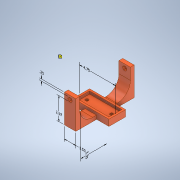
# Autodesk Inventor part: connectorToTubeBrackeCradleTmp
Saved by Autodesk Inventor 2022 (Build 260153070, 153G)
## iProperties
Created: 2020-07-23
Part Number: connectorToTubeBrackeCradleTmp
Material: PBT Plastic
Document SubType Name: Modeling
Designer: robst
Density: 1.31 g/cm^3
Appearance: Smooth - Light Orange
Mass: 391.418 g
Surface Area: 592.905 cm^2
Volume: 298.793 cm^3
Author: robst
Autodesk Inventor part; units mm, degrees
(part 1 of 3)
ref_plane "YZ Plane" through (0, 0, 0) normal (1, 0, 0) x (0, 1, 0)
ref_plane "XZ Plane" through (0, 0, 0) normal (0, 1, 0) x (-1, 0, 0)
ref_plane "XY Plane" through (0, 0, 0) normal (0, 0, 1) x (1, 0, 0)
sketch "Sketch1" plane through (0, 0, 0) normal (0, 1, 0) x (-1, 0, 0)
  line L0 (53.975, 21.59) -> (-53.975, 21.59)
  line L1 (-53.975, 21.59) -> (-53.975, -21.59)
  line L2 (-53.975, -21.59) -> (53.975, -21.59)
  line L3 (53.975, -21.59) -> (53.975, 21.59)
  line L4 (53.975, 21.59) -> (-53.975, -21.59) construction
  line L5 (-53.975, 21.59) -> (53.975, -21.59) construction
  line L6 (60.325, 27.94) -> (-60.325, 27.94)
  line L7 (-60.325, 27.94) -> (-60.325, -27.94)
  line L8 (-60.325, -27.94) -> (60.325, -27.94)
  line L9 (60.325, -27.94) -> (60.325, 27.94)
  line L10 (60.325, 27.94) -> (-60.325, -27.94) construction
  line L11 (-60.325, 27.94) -> (60.325, -27.94) construction
  point P0 (0, 0)
  dimension "d0" = 43.18
  dimension "d1" = 107.95
  dimension "d2" = 6.35
  dimension "d3" = 6.35
  constraints: 24 end point, 4 midpoint, 4 parallel, 2 horizontal, 2 perpendicular
  measures "d0" distance of L0.end L1.end
  measures "d1" distance between parallel lines of L1 L3
  measures "d2" distance between parallel lines of L8 L2
  measures "d3" distance between parallel lines of L9 L3
extrude "Extrusion1" add sketch "Sketch1" against normal blind 12.065 contours L3 L2 L1 L0 | L9 L8 L7 L6
extrude "Extrusion2" add sketch "Sketch1" along normal blind 8.89
sketch "Sketch2" plane through (0, 0, 0) normal (0, 1, 0) x (1, 0, 0)
  line L0 (-53.975, 21.59) -> (-53.975, -21.59) construction
  line L1 (-53.975, 0) -> (53.975, 0) construction
  line L2 (53.975, -21.59) -> (53.975, 21.59) construction
  point P0 (0, 0)
  point P1 (-41.275, 0)
  point P2 (41.275, 0)
  dimension "d8" = 12.7
  dimension "d9" = 12.7
  constraints: 2 end point, 2 midpoint, 2 point on line
  measures "d8" distance from line of point (-41.275, 0) L0
  measures "d9" distance from line of point (41.275, 0) L2
hole "Hole1" at (-41.275, 0, 0) at (41.275, 0, 0) direction (0, -1, 0) diameter 5.1054 end through all counterbore diameter 10.16 counterbore depth 2.54 clearance for "Hex Machine Screw" size "#10" standard "Ansi Unified Screw Threads"
sketch "Sketch15" plane through (-60.325, -12.065, 27.94) normal (0, 0, 1) x (1, 0, 0)
  line L0 (0, 20.955) -> (120.65, 20.955) projected
  line L1 (120.65, 20.955) -> (120.65, 0) projected
  line L2 (120.65, 0) -> (0, 0) projected
  line L3 (0, 0) -> (0, 20.955) projected
  line L4 (0, 20.955) -> (120.65, 0) construction
  line L5 (0, 0) -> (120.65, 20.955) construction
  line L6 (41.275, 0) -> (79.375, 0)
  line L7 (79.375, 0) -> (79.375, 20.955)
  line L8 (79.375, 20.955) -> (41.275, 20.955)
  line L9 (41.275, 20.955) -> (41.275, 0)
  line L10 (41.275, 0) -> (79.375, 20.955) construction
  line L11 (79.375, 0) -> (41.275, 20.955) construction
  line L12 (114.3, 12.065) -> (6.35, 12.065) projected
  point P0 (60.325, 12.065)
  point P1 (60.325, 10.4775)
  point P2 (79.375, 12.065)
  point P3 (41.275, 12.065)
  point P4 (41.275, 0)
  point P5 (79.375, 0)
  dimension "d109" = 38.1
  constraints: 16 end point, 3 midpoint, 3 parallel, 1 collinear, 1 perpendicular
  measures "d109" distance between parallel lines of L7 L9
extrude "Extrusion10" add sketch "Sketch15" along normal blind 69.85 contours L12 L7 L2 L9
sketch "Sketch16" plane through (-19.05, 0, 27.94) normal (0, 1, 0) x (1, 0, 0)
  line L0 (0, -69.85) -> (38.1, -69.85) projected
  line L1 (38.1, 0) -> (38.1, -69.85) projected
  line L2 (0, -69.85) -> (38.1, -69.85)
  line L3 (38.1, -69.85) -> (38.1, -57.15)
  line L4 (38.1, -57.15) -> (0, -57.15)
  line L5 (0, -57.15) -> (0, -69.85)
  point P0 (19.05, 27.94)
  dimension "d103" = 12.7
  constraints: 8 end point, 2 parallel, 1 horizontal, 1 perpendicular, 1 point on line
  measures "d103" distance between parallel lines of L4 L0
extrude "Extrusion11" add sketch "Sketch16" along normal blind 82.55
sketch "Sketch17" plane through (-60.325, -12.065, 97.79) normal (0, 0, 1) x (1, 0, 0)
  line L0 (41.275, 94.615) -> (79.375, 94.615) construction
  line L1 (41.275, 0) -> (79.375, 0) construction
  line L2 (79.375, 94.615) -> (41.275, 94.615) construction
  line L3 (60.325, 94.615) -> (60.325, 0) construction
  line L4 (67.804, 81.915) -> (64.0645, 75.438)
  line L5 (64.0645, 75.438) -> (56.5855, 75.438)
  line L6 (56.5855, 75.438) -> (52.846, 81.915)
  line L7 (52.846, 81.915) -> (56.5855, 88.392)
  line L8 (56.5855, 88.392) -> (64.0645, 88.392)
  line L9 (64.0645, 88.392) -> (67.804, 81.915)
  point P0 (60.325, 12.065)
  point P1 (60.325, 81.915)
  dimension "d119" = 12.7
  dimension "d120" = 12.954
  constraints: 14 end point, 2 midpoint, 1 horizontal, 1 point on line, 13 other
  measures "d119" distance from line of point (60.325, 81.915) L0
  measures "d120" distance between parallel lines of L5 L8
extrude "Extrusion12" cut sketch "Sketch17" against normal through all
mirror "Mirror8" about plane through (0, 0, 0) normal (0, 0, 1) of "Extrusion11", "Extrusion12", "Extrusion10"
fillet "Fillet1" radius 44.45 2 edges at (0, 0, -85.09) (0, 0, 85.09)
sketch "Sketch18" plane through (0, -12.065, 0) normal (0, -1, 0) x (1, 0, 0)
  line L0 (-19.05, 97.79) -> (19.05, 97.79) construction
  line L1 (0, 97.79) -> (0, -97.79) construction
  line L2 (-19.05, -97.79) -> (19.05, -97.79) construction
  line L3 (-6.35, -88.0484) -> (-6.35, -88.8511)
  line L4 (-6.35, -88.8511) -> (-6.8337, -88.8511)
  spline S0 degree 2 poles (-6.8337, -88.8511) (-6.6793, -89.0364) (-6.4735, -89.3091) (-6.386, -89.4943) knots 0 0 0 1 2 2 2
  spline S1 degree 2 poles (-6.386, -89.4943) (-6.3037, -89.6642) (-6.2162, -90.0295) (-6.2162, -90.2714) knots 0 0 0 1 2 2 2
  spline S2 degree 2 poles (-6.2162, -90.2714) (-6.2162, -90.6625) (-6.5404, -91.3211) (-6.8543, -91.5527) knots 0 0 0 1 2 2 2
  spline S3 degree 2 poles (-6.8543, -91.5527) (-7.1682, -91.7843) (-8.0944, -92.0415) (-8.6965, -92.0415) knots 0 0 0 1 2 2 2
  spline S4 degree 2 poles (-8.6965, -92.0415) (-9.3243, -92.0415) (-10.2403, -91.7174) (-10.585, -91.4343) knots 0 0 0 1 2 2 2
  spline S5 degree 2 poles (-10.585, -91.4343) (-10.8938, -91.1719) (-11.2489, -90.436) (-11.2489, -90.0295) knots 0 0 0 1 2 2 2
  spline S6 degree 2 poles (-11.2489, -90.0295) (-11.2489, -89.6744) (-11.0893, -89.1444) (-10.9247, -88.8511) knots 0 0 0 1 2 2 2
  line L5 (-10.9247, -88.8511) -> (-12.983, -88.8511)
  line L6 (-12.983, -88.8511) -> (-12.983, -88.0484)
  line L7 (-12.983, -88.0484) -> (-6.35, -88.0484)
  line L8 (-7.5078, -88.8511) -> (-10.2609, -88.8511)
  spline S7 degree 2 poles (-10.2609, -88.8511) (-10.4049, -89.1496) (-10.513, -89.623) (-10.513, -89.8957) knots 0 0 0 1 2 2 2
  spline S8 degree 2 poles (-10.513, -89.8957) (-10.513, -90.5132) (-9.5868, -91.2131) (-8.712, -91.2131) knots 0 0 0 1 2 2 2
  spline S9 degree 2 poles (-8.712, -91.2131) (-7.868, -91.2131) (-6.9778, -90.6779) (-6.9778, -90.0861) knots 0 0 0 1 2 2 2
  spline S10 degree 2 poles (-6.9778, -90.0861) (-6.9778, -89.7722) (-7.266, -89.1341) (-7.5078, -88.8511) knots 0 0 0 1 2 2 2
  line L9 (-6.35, -86.0672) -> (-6.35, -86.8699)
  line L10 (-6.35, -86.8699) -> (-11.1151, -86.8699)
  line L11 (-11.1151, -86.8699) -> (-11.1151, -86.0672)
  line L12 (-11.1151, -86.0672) -> (-6.35, -86.0672)
  line L13 (-11.9075, -86.0106) -> (-11.9075, -86.9214)
  line L14 (-11.9075, -86.9214) -> (-12.7412, -86.9214)
  line L15 (-12.7412, -86.9214) -> (-12.7412, -86.0106)
  line L16 (-12.7412, -86.0106) -> (-11.9075, -86.0106)
  line L17 (-10.2557, -82.3622) -> (-10.2557, -82.4033)
  spline S11 degree 2 poles (-10.2557, -82.4033) (-10.2814, -82.496) (-10.2917, -82.6966) (-10.2917, -82.8356) knots 0 0 0 1 2 2 2
  spline S12 degree 2 poles (-10.2917, -82.8356) (-10.2917, -83.1598) (-10.0087, -83.7979) (-9.7308, -84.086) knots 0 0 0 1 2 2 2
  line L18 (-9.7308, -84.086) -> (-6.35, -84.086)
  line L19 (-6.35, -84.086) -> (-6.35, -84.8888)
  line L20 (-6.35, -84.8888) -> (-11.1151, -84.8888)
  line L21 (-11.1151, -84.8888) -> (-11.1151, -84.086)
  line L22 (-11.1151, -84.086) -> (-10.4049, -84.086)
  spline S13 degree 2 poles (-10.4049, -84.086) (-10.796, -83.6486) (-11.1151, -82.9951) (-11.1151, -82.6864) knots 0 0 0 1 2 2 2
  spline S14 degree 2 poles (-11.1151, -82.6864) (-11.1151, -82.5629) (-11.1048, -82.4394) (-11.0893, -82.3622) knots 0 0 0 1 2 2 2
  line L23 (-11.0893, -82.3622) -> (-10.2557, -82.3622)
  line L24 (-6.35, -80.2678) -> (-6.35, -81.2867)
  line L25 (-6.35, -81.2867) -> (-7.5644, -81.2867)
  line L26 (-7.5644, -81.2867) -> (-7.5644, -80.2678)
  line L27 (-7.5644, -80.2678) -> (-6.35, -80.2678)
  line L28 (-9.9006, -80.2678) -> (-9.9006, -81.2867)
  line L29 (-9.9006, -81.2867) -> (-11.1151, -81.2867)
  line L30 (-11.1151, -81.2867) -> (-11.1151, -80.2678)
  line L31 (-11.1151, -80.2678) -> (-9.9006, -80.2678)
  line L32 (-6.35, -74.3809) -> (-11.9487, -74.3809)
  line L33 (-11.9487, -74.3809) -> (-11.9487, -76.5113)
  line L34 (-11.9487, -76.5113) -> (-12.7, -76.5113)
  line L35 (-12.7, -76.5113) -> (-12.7, -71.4066)
  line L36 (-12.7, -71.4066) -> (-11.9487, -71.4066)
  line L37 (-11.9487, -71.4066) -> (-11.9487, -73.537)
  line L38 (-11.9487, -73.537) -> (-6.35, -73.537)
  line L39 (-6.35, -73.537) -> (-6.35, -74.3809)
  spline S15 degree 2 poles (-6.2419, -68.7514) (-6.2419, -69.8937) (-7.5233, -71.1493) (-8.7068, -71.1493) knots 0 0 0 1 2 2 2
  spline S16 degree 2 poles (-8.7068, -71.1493) (-9.8698, -71.1493) (-11.2489, -69.9298) (-11.2489, -68.9469) knots 0 0 0 1 2 2 2
  spline S17 degree 2 poles (-11.2489, -68.9469) (-11.2489, -68.5043) (-10.9916, -67.8199) (-10.7188, -67.5678) knots 0 0 0 1 2 2 2
  spline S18 degree 2 poles (-10.7188, -67.5678) (-10.4461, -67.3105) (-9.6588, -67.0378) (-9.0876, -67.0378) knots 0 0 0 1 2 2 2
  line L40 (-9.0876, -67.0378) -> (-8.6502, -67.0378)
  line L41 (-8.6502, -67.0378) -> (-8.6502, -70.3363)
  spline S19 degree 2 poles (-8.6502, -70.3363) (-7.8217, -70.3363) (-6.9418, -69.5026) (-6.9418, -68.7616) knots 0 0 0 1 2 2 2
  spline S20 degree 2 poles (-6.9418, -68.7616) (-6.9418, -68.4992) (-7.0601, -67.9898) (-7.1528, -67.7839) knots 0 0 0 1 2 2 2
  spline S21 degree 2 poles (-7.1528, -67.7839) (-7.2557, -67.5678) (-7.4358, -67.2693) (-7.5181, -67.1716) knots 0 0 0 1 2 2 2
  line L42 (-7.5181, -67.1716) -> (-7.5181, -67.1253)
  line L43 (-7.5181, -67.1253) -> (-6.6433, -67.1253)
  spline S22 degree 2 poles (-6.6433, -67.1253) (-6.5867, -67.2642) (-6.422, -67.6862) (-6.3757, -67.8508) knots 0 0 0 1 2 2 2
  spline S23 degree 2 poles (-6.3757, -67.8508) (-6.3088, -68.0824) (-6.2419, -68.4632) (-6.2419, -68.7514) knots 0 0 0 1 2 2 2
  spline S24 degree 2 poles (-9.2626, -67.8199) (-9.5868, -67.8302) (-10.0602, -67.964) (-10.2197, -68.0927) knots 0 0 0 1 2 2 2
  spline S25 degree 2 poles (-10.2197, -68.0927) (-10.3998, -68.2316) (-10.5902, -68.669) (-10.5902, -68.9932) knots 0 0 0 1 2 2 2
  spline S26 degree 2 poles (-10.5902, -68.9932) (-10.5902, -69.3123) (-10.3998, -69.7599) (-10.2145, -69.9452) knots 0 0 0 1 2 2 2
  spline S27 degree 2 poles (-10.2145, -69.9452) (-10.0241, -70.1253) (-9.5662, -70.3105) (-9.2626, -70.3363) knots 0 0 0 1 2 2 2
  line L44 (-9.2626, -70.3363) -> (-9.2626, -67.8199)
  line L45 (-6.35, -65.4065) -> (-6.35, -66.2093)
  line L46 (-6.35, -66.2093) -> (-12.983, -66.2093)
  line L47 (-12.983, -66.2093) -> (-12.983, -65.4065)
  line L48 (-12.983, -65.4065) -> (-6.35, -65.4065)
  spline S28 degree 2 poles (-6.2419, -62.1595) (-6.2419, -63.3019) (-7.5233, -64.5575) (-8.7068, -64.5575) knots 0 0 0 1 2 2 2
  spline S29 degree 2 poles (-8.7068, -64.5575) (-9.8698, -64.5575) (-11.2489, -63.3379) (-11.2489, -62.355) knots 0 0 0 1 2 2 2
  spline S30 degree 2 poles (-11.2489, -62.355) (-11.2489, -61.9125) (-10.9916, -61.2281) (-10.7188, -60.9759) knots 0 0 0 1 2 2 2
  spline S31 degree 2 poles (-10.7188, -60.9759) (-10.4461, -60.7187) (-9.6588, -60.4459) (-9.0876, -60.4459) knots 0 0 0 1 2 2 2
  line L49 (-9.0876, -60.4459) -> (-8.6502, -60.4459)
  line L50 (-8.6502, -60.4459) -> (-8.6502, -63.7444)
  spline S32 degree 2 poles (-8.6502, -63.7444) (-7.8217, -63.7444) (-6.9418, -62.9108) (-6.9418, -62.1698) knots 0 0 0 1 2 2 2
  spline S33 degree 2 poles (-6.9418, -62.1698) (-6.9418, -61.9073) (-7.0601, -61.3979) (-7.1528, -61.1921) knots 0 0 0 1 2 2 2
  spline S34 degree 2 poles (-7.1528, -61.1921) (-7.2557, -60.9759) (-7.4358, -60.6775) (-7.5181, -60.5797) knots 0 0 0 1 2 2 2
  line L51 (-7.5181, -60.5797) -> (-7.5181, -60.5334)
  line L52 (-7.5181, -60.5334) -> (-6.6433, -60.5334)
  spline S35 degree 2 poles (-6.6433, -60.5334) (-6.5867, -60.6723) (-6.422, -61.0943) (-6.3757, -61.259) knots 0 0 0 1 2 2 2
  spline S36 degree 2 poles (-6.3757, -61.259) (-6.3088, -61.4905) (-6.2419, -61.8713) (-6.2419, -62.1595) knots 0 0 0 1 2 2 2
  spline S37 degree 2 poles (-9.2626, -61.2281) (-9.5868, -61.2384) (-10.0602, -61.3722) (-10.2197, -61.5008) knots 0 0 0 1 2 2 2
  spline S38 degree 2 poles (-10.2197, -61.5008) (-10.3998, -61.6398) (-10.5902, -62.0772) (-10.5902, -62.4014) knots 0 0 0 1 2 2 2
  spline S39 degree 2 poles (-10.5902, -62.4014) (-10.5902, -62.7204) (-10.3998, -63.1681) (-10.2145, -63.3533) knots 0 0 0 1 2 2 2
  spline S40 degree 2 poles (-10.2145, -63.3533) (-10.0241, -63.5334) (-9.5662, -63.7187) (-9.2626, -63.7444) knots 0 0 0 1 2 2 2
  line L53 (-9.2626, -63.7444) -> (-9.2626, -61.2281)
  spline S41 degree 2 poles (-6.2368, -58.3464) (-6.2368, -58.825) (-6.4941, -59.6535) (-6.6382, -59.9262) knots 0 0 0 1 2 2 2
  line L54 (-6.6382, -59.9262) -> (-7.5387, -59.9262)
  line L55 (-7.5387, -59.9262) -> (-7.5387, -59.885)
  spline S42 degree 2 poles (-7.5387, -59.885) (-7.4564, -59.7821) (-7.2608, -59.5042) (-7.1528, -59.2727) knots 0 0 0 1 2 2 2
  spline S43 degree 2 poles (-7.1528, -59.2727) (-7.055, -59.072) (-6.9109, -58.578) (-6.9109, -58.3155) knots 0 0 0 1 2 2 2
  spline S44 degree 2 poles (-6.9109, -58.3155) (-6.9109, -58.1251) (-6.9984, -57.6877) (-7.0704, -57.5848) knots 0 0 0 1 2 2 2
  spline S45 degree 2 poles (-7.0704, -57.5848) (-7.1682, -57.4356) (-7.3895, -57.3018) (-7.6159, -57.3018) knots 0 0 0 1 2 2 2
  spline S46 degree 2 poles (-7.6159, -57.3018) (-7.8989, -57.3018) (-8.1922, -57.6105) (-8.29, -58.0068) knots 0 0 0 1 2 2 2
  spline S47 degree 2 poles (-8.29, -58.0068) (-8.326, -58.1612) (-8.4289, -58.6552) (-8.4855, -58.8661) knots 0 0 0 1 2 2 2
  spline S48 degree 2 poles (-8.4855, -58.8661) (-8.6451, -59.4116) (-9.3037, -59.9056) (-9.772, -59.9056) knots 0 0 0 1 2 2 2
  spline S49 degree 2 poles (-9.772, -59.9056) (-10.4204, -59.9056) (-11.2283, -58.933) (-11.2283, -58.1303) knots 0 0 0 1 2 2 2
  spline S50 degree 2 poles (-11.2283, -58.1303) (-11.2283, -57.7341) (-11.0327, -56.9313) (-10.8835, -56.6586) knots 0 0 0 1 2 2 2
  line L56 (-10.8835, -56.6586) -> (-10.0241, -56.6586)
  line L57 (-10.0241, -56.6586) -> (-10.0241, -56.6997)
  spline S51 degree 2 poles (-10.0241, -56.6997) (-10.2712, -57.0085) (-10.5542, -57.7598) (-10.5542, -58.1457) knots 0 0 0 1 2 2 2
  spline S52 degree 2 poles (-10.5542, -58.1457) (-10.5542, -58.542) (-10.2197, -59.0874) (-9.8852, -59.0874) knots 0 0 0 1 2 2 2
  spline S53 degree 2 poles (-9.8852, -59.0874) (-9.5816, -59.0874) (-9.2883, -58.7632) (-9.1957, -58.403) knots 0 0 0 1 2 2 2
  spline S54 degree 2 poles (-9.1957, -58.403) (-9.1494, -58.2281) (-9.0567, -57.7855) (-9.0001, -57.5437) knots 0 0 0 1 2 2 2
  spline S55 degree 2 poles (-9.0001, -57.5437) (-8.8663, -57.0188) (-8.254, -56.4836) (-7.7239, -56.4836) knots 0 0 0 1 2 2 2
  spline S56 degree 2 poles (-7.7239, -56.4836) (-7.4152, -56.4836) (-6.8697, -56.7255) (-6.669, -56.9622) knots 0 0 0 1 2 2 2
  spline S57 degree 2 poles (-6.669, -56.9622) (-6.4581, -57.2143) (-6.2368, -57.8576) (-6.2368, -58.3464) knots 0 0 0 1 2 2 2
  spline S58 degree 2 poles (-6.2419, -53.8438) (-6.2419, -54.3378) (-6.5455, -55.156) (-6.8543, -55.4493) knots 0 0 0 1 2 2 2
  spline S59 degree 2 poles (-6.8543, -55.4493) (-7.1579, -55.7426) (-8.0944, -56.0668) (-8.7222, -56.0668) knots 0 0 0 1 2 2 2
  spline S60 degree 2 poles (-8.7222, -56.0668) (-9.35, -56.0668) (-10.266, -55.7323) (-10.5748, -55.4493) knots 0 0 0 1 2 2 2
  spline S61 degree 2 poles (-10.5748, -55.4493) (-10.8887, -55.1663) (-11.2231, -54.3275) (-11.2231, -53.8438) knots 0 0 0 1 2 2 2
  spline S62 degree 2 poles (-11.2231, -53.8438) (-11.2231, -53.4527) (-11.0019, -52.722) (-10.8578, -52.439) knots 0 0 0 1 2 2 2
  line L58 (-10.8578, -52.439) -> (-9.9573, -52.439)
  line L59 (-9.9573, -52.439) -> (-9.9573, -52.4853)
  spline S63 degree 2 poles (-9.9573, -52.4853) (-10.0293, -52.5727) (-10.2145, -52.8403) (-10.3123, -53.0307) knots 0 0 0 1 2 2 2
  spline S64 degree 2 poles (-10.3123, -53.0307) (-10.3947, -53.2005) (-10.5233, -53.6534) (-10.5233, -53.8592) knots 0 0 0 1 2 2 2
  spline S65 degree 2 poles (-10.5233, -53.8592) (-10.5233, -54.4819) (-9.5816, -55.2383) (-8.7222, -55.2383) knots 0 0 0 1 2 2 2
  spline S66 degree 2 poles (-8.7222, -55.2383) (-7.8835, -55.2383) (-6.9418, -54.5076) (-6.9418, -53.8592) knots 0 0 0 1 2 2 2
  spline S67 degree 2 poles (-6.9418, -53.8592) (-6.9418, -53.4681) (-7.266, -52.758) (-7.5181, -52.4853) knots 0 0 0 1 2 2 2
  line L60 (-7.5181, -52.4853) -> (-7.5181, -52.439)
  line L61 (-7.5181, -52.439) -> (-6.6176, -52.439)
  spline S68 degree 2 poles (-6.6176, -52.439) (-6.561, -52.5573) (-6.4015, -52.9175) (-6.3654, -53.0616) knots 0 0 0 1 2 2 2
  spline S69 degree 2 poles (-6.3654, -53.0616) (-6.3037, -53.2674) (-6.2419, -53.5916) (-6.2419, -53.8438) knots 0 0 0 1 2 2 2
  spline S70 degree 2 poles (-8.7325, -47.7922) (-7.5284, -47.7922) (-6.2162, -48.9501) (-6.2162, -49.9175) knots 0 0 0 1 2 2 2
  spline S71 degree 2 poles (-6.2162, -49.9175) (-6.2162, -50.9106) (-7.5696, -52.0479) (-8.7325, -52.0479) knots 0 0 0 1 2 2 2
  spline S72 degree 2 poles (-8.7325, -52.0479) (-9.9264, -52.0479) (-11.2489, -50.8746) (-11.2489, -49.9175) knots 0 0 0 1 2 2 2
  spline S73 degree 2 poles (-11.2489, -49.9175) (-11.2489, -48.9501) (-9.9315, -47.7922) (-8.7325, -47.7922) knots 0 0 0 1 2 2 2
  spline S74 degree 2 poles (-8.7325, -48.6207) (-9.6588, -48.6207) (-10.5593, -49.2948) (-10.5593, -49.9175) knots 0 0 0 1 2 2 2
  spline S75 degree 2 poles (-10.5593, -49.9175) (-10.5593, -50.5401) (-9.6588, -51.2194) (-8.7325, -51.2194) knots 0 0 0 1 2 2 2
  spline S76 degree 2 poles (-8.7325, -51.2194) (-7.832, -51.2194) (-6.9058, -50.5401) (-6.9058, -49.9175) knots 0 0 0 1 2 2 2
  spline S77 degree 2 poles (-6.9058, -49.9175) (-6.9058, -49.3) (-7.8166, -48.6207) (-8.7325, -48.6207) knots 0 0 0 1 2 2 2
  spline S78 degree 2 poles (-8.8612, -42.9757) (-7.6673, -42.9757) (-6.2574, -44.1129) (-6.2574, -44.9826) knots 0 0 0 1 2 2 2
  spline S79 degree 2 poles (-6.2574, -44.9826) (-6.2574, -45.3377) (-6.422, -45.8831) (-6.5919, -46.1661) knots 0 0 0 1 2 2 2
  line L62 (-6.5919, -46.1661) -> (-4.5953, -46.1661)
  line L63 (-4.5953, -46.1661) -> (-4.5953, -46.9689)
  line L64 (-4.5953, -46.9689) -> (-11.1151, -46.9689)
  line L65 (-11.1151, -46.9689) -> (-11.1151, -46.1661)
  line L66 (-11.1151, -46.1661) -> (-10.6159, -46.1661)
  spline S80 degree 2 poles (-10.6159, -46.1661) (-10.8887, -45.8677) (-11.2489, -45.137) (-11.2489, -44.7099) knots 0 0 0 1 2 2 2
  spline S81 degree 2 poles (-11.2489, -44.7099) (-11.2489, -43.8917) (-9.9521, -42.9757) (-8.8612, -42.9757) knots 0 0 0 1 2 2 2
  spline S82 degree 2 poles (-8.7686, -43.8042) (-9.5868, -43.8042) (-10.4873, -44.3239) (-10.4873, -44.9054) knots 0 0 0 1 2 2 2
  spline S83 degree 2 poles (-10.4873, -44.9054) (-10.4873, -45.245) (-10.1837, -45.8831) (-9.947, -46.1661) knots 0 0 0 1 2 2 2
  line L67 (-9.947, -46.1661) -> (-7.2402, -46.1661)
  spline S84 degree 2 poles (-7.2402, -46.1661) (-7.091, -45.8522) (-6.9778, -45.4046) (-6.9778, -45.1164) knots 0 0 0 1 2 2 2
  spline S85 degree 2 poles (-6.9778, -45.1164) (-6.9778, -44.4937) (-7.8938, -43.8042) (-8.7686, -43.8042) knots 0 0 0 1 2 2 2
  spline S86 degree 2 poles (-6.2419, -40.0734) (-6.2419, -41.2158) (-7.5233, -42.4714) (-8.7068, -42.4714) knots 0 0 0 1 2 2 2
  spline S87 degree 2 poles (-8.7068, -42.4714) (-9.8698, -42.4714) (-11.2489, -41.2518) (-11.2489, -40.269) knots 0 0 0 1 2 2 2
  spline S88 degree 2 poles (-11.2489, -40.269) (-11.2489, -39.8264) (-10.9916, -39.142) (-10.7188, -38.8899) knots 0 0 0 1 2 2 2
  spline S89 degree 2 poles (-10.7188, -38.8899) (-10.4461, -38.6326) (-9.6588, -38.3599) (-9.0876, -38.3599) knots 0 0 0 1 2 2 2
  line L68 (-9.0876, -38.3599) -> (-8.6502, -38.3599)
  line L69 (-8.6502, -38.3599) -> (-8.6502, -41.6584)
  spline S90 degree 2 poles (-8.6502, -41.6584) (-7.8217, -41.6584) (-6.9418, -40.8247) (-6.9418, -40.0837) knots 0 0 0 1 2 2 2
  spline S91 degree 2 poles (-6.9418, -40.0837) (-6.9418, -39.8213) (-7.0601, -39.3118) (-7.1528, -39.106) knots 0 0 0 1 2 2 2
  spline S92 degree 2 poles (-7.1528, -39.106) (-7.2557, -38.8899) (-7.4358, -38.5914) (-7.5181, -38.4937) knots 0 0 0 1 2 2 2
  line L70 (-7.5181, -38.4937) -> (-7.5181, -38.4473)
  line L71 (-7.5181, -38.4473) -> (-6.6433, -38.4473)
  spline S93 degree 2 poles (-6.6433, -38.4473) (-6.5867, -38.5863) (-6.422, -39.0082) (-6.3757, -39.1729) knots 0 0 0 1 2 2 2
  spline S94 degree 2 poles (-6.3757, -39.1729) (-6.3088, -39.4045) (-6.2419, -39.7853) (-6.2419, -40.0734) knots 0 0 0 1 2 2 2
  spline S95 degree 2 poles (-9.2626, -39.142) (-9.5868, -39.1523) (-10.0602, -39.2861) (-10.2197, -39.4148) knots 0 0 0 1 2 2 2
  spline S96 degree 2 poles (-10.2197, -39.4148) (-10.3998, -39.5537) (-10.5902, -39.9911) (-10.5902, -40.3153) knots 0 0 0 1 2 2 2
  spline S97 degree 2 poles (-10.5902, -40.3153) (-10.5902, -40.6343) (-10.3998, -41.082) (-10.2145, -41.2673) knots 0 0 0 1 2 2 2
  spline S98 degree 2 poles (-10.2145, -41.2673) (-10.0241, -41.4474) (-9.5662, -41.6326) (-9.2626, -41.6584) knots 0 0 0 1 2 2 2
  line L72 (-9.2626, -41.6584) -> (-9.2626, -39.142)
  spline S99 degree 2 poles (-10.7857, -33.4713) (-10.3741, -33.4713) (-9.6331, -33.7646) (-9.3758, -34.027) knots 0 0 0 1 2 2 2
  spline S100 degree 2 poles (-9.3758, -34.027) (-9.0516, -34.3564) (-8.7171, -35.2466) (-8.7171, -35.9259) knots 0 0 0 1 2 2 2
  line L73 (-8.7171, -35.9259) -> (-8.7171, -36.6411)
  line L74 (-8.7171, -36.6411) -> (-6.35, -36.6411)
  line L75 (-6.35, -36.6411) -> (-6.35, -37.4851)
  line L76 (-6.35, -37.4851) -> (-12.7, -37.4851)
  line L77 (-12.7, -37.4851) -> (-12.7, -35.8898)
  spline S101 degree 2 poles (-12.7, -35.8898) (-12.7, -35.3238) (-12.5147, -34.5313) (-12.3038, -34.2277) knots 0 0 0 1 2 2 2
  spline S102 degree 2 poles (-12.3038, -34.2277) (-12.0619, -33.8727) (-11.3158, -33.4713) (-10.7857, -33.4713) knots 0 0 0 1 2 2 2
  spline S103 degree 2 poles (-10.76, -34.3512) (-11.0893, -34.3512) (-11.5731, -34.5776) (-11.7274, -34.8092) knots 0 0 0 1 2 2 2
  spline S104 degree 2 poles (-11.7274, -34.8092) (-11.8612, -35.0099) (-11.9693, -35.5451) (-11.9693, -35.9413) knots 0 0 0 1 2 2 2
  line L78 (-11.9693, -35.9413) -> (-11.9693, -36.6411)
  line L79 (-11.9693, -36.6411) -> (-9.4375, -36.6411)
  line L80 (-9.4375, -36.6411) -> (-9.4375, -36.0648)
  spline S105 degree 2 poles (-9.4375, -36.0648) (-9.4375, -35.5502) (-9.6022, -34.9173) (-9.8183, -34.7114) knots 0 0 0 1 2 2 2
  spline S106 degree 2 poles (-9.8183, -34.7114) (-10.0087, -34.521) (-10.4564, -34.3512) (-10.76, -34.3512) knots 0 0 0 1 2 2 2
  line L81 (-10.2557, -30.2037) -> (-10.2557, -30.2448)
  spline S107 degree 2 poles (-10.2557, -30.2448) (-10.2814, -30.3375) (-10.2917, -30.5381) (-10.2917, -30.6771) knots 0 0 0 1 2 2 2
  spline S108 degree 2 poles (-10.2917, -30.6771) (-10.2917, -31.0013) (-10.0087, -31.6394) (-9.7308, -31.9275) knots 0 0 0 1 2 2 2
  line L82 (-9.7308, -31.9275) -> (-6.35, -31.9275)
  line L83 (-6.35, -31.9275) -> (-6.35, -32.7303)
  line L84 (-6.35, -32.7303) -> (-11.1151, -32.7303)
  line L85 (-11.1151, -32.7303) -> (-11.1151, -31.9275)
  line L86 (-11.1151, -31.9275) -> (-10.4049, -31.9275)
  spline S109 degree 2 poles (-10.4049, -31.9275) (-10.796, -31.4901) (-11.1151, -30.8366) (-11.1151, -30.5279) knots 0 0 0 1 2 2 2
  spline S110 degree 2 poles (-11.1151, -30.5279) (-11.1151, -30.4044) (-11.1048, -30.2808) (-11.0893, -30.2037) knots 0 0 0 1 2 2 2
  line L87 (-11.0893, -30.2037) -> (-10.2557, -30.2037)
  spline S111 degree 2 poles (-8.7325, -25.665) (-7.5284, -25.665) (-6.2162, -26.8228) (-6.2162, -27.7903) knots 0 0 0 1 2 2 2
  spline S112 degree 2 poles (-6.2162, -27.7903) (-6.2162, -28.7834) (-7.5696, -29.9206) (-8.7325, -29.9206) knots 0 0 0 1 2 2 2
  spline S113 degree 2 poles (-8.7325, -29.9206) (-9.9264, -29.9206) (-11.2489, -28.7474) (-11.2489, -27.7903) knots 0 0 0 1 2 2 2
  spline S114 degree 2 poles (-11.2489, -27.7903) (-11.2489, -26.8228) (-9.9315, -25.665) (-8.7325, -25.665) knots 0 0 0 1 2 2 2
  spline S115 degree 2 poles (-8.7325, -26.4935) (-9.6588, -26.4935) (-10.5593, -27.1676) (-10.5593, -27.7903) knots 0 0 0 1 2 2 2
  spline S116 degree 2 poles (-10.5593, -27.7903) (-10.5593, -28.4129) (-9.6588, -29.0922) (-8.7325, -29.0922) knots 0 0 0 1 2 2 2
  spline S117 degree 2 poles (-8.7325, -29.0922) (-7.832, -29.0922) (-6.9058, -28.4129) (-6.9058, -27.7903) knots 0 0 0 1 2 2 2
  spline S118 degree 2 poles (-6.9058, -27.7903) (-6.9058, -27.1727) (-7.8166, -26.4935) (-8.7325, -26.4935) knots 0 0 0 1 2 2 2
  spline S119 degree 2 poles (-6.2162, -23.5449) (-5.4032, -23.5449) (-4.5489, -24.4197) (-4.5489, -25.1864) knots 0 0 0 1 2 2 2
  spline S120 degree 2 poles (-4.5489, -25.1864) (-4.5489, -25.3202) (-4.5747, -25.6496) (-4.6004, -25.8091) knots 0 0 0 1 2 2 2
  line L88 (-4.6004, -25.8091) -> (-5.3208, -25.8091)
  line L89 (-5.3208, -25.8091) -> (-5.3208, -25.7628)
  spline S121 degree 2 poles (-5.3208, -25.7628) (-5.3002, -25.6702) (-5.2591, -25.4437) (-5.2591, -25.3408) knots 0 0 0 1 2 2 2
  spline S122 degree 2 poles (-5.2591, -25.3408) (-5.2591, -25.0218) (-5.4186, -24.605) (-5.5884, -24.5072) knots 0 0 0 1 2 2 2
  spline S123 degree 2 poles (-5.5884, -24.5072) (-5.7428, -24.4094) (-6.2111, -24.3477) (-6.5455, -24.3477) knots 0 0 0 1 2 2 2
  line L90 (-6.5455, -24.3477) -> (-10.4513, -24.3477)
  line L91 (-10.4513, -24.3477) -> (-10.4513, -25.207)
  line L92 (-10.4513, -25.207) -> (-11.1151, -25.207)
  line L93 (-11.1151, -25.207) -> (-11.1151, -23.5449)
  line L94 (-11.1151, -23.5449) -> (-6.2162, -23.5449)
  line L95 (-11.9075, -23.5398) -> (-11.9075, -24.4506)
  line L96 (-11.9075, -24.4506) -> (-12.7412, -24.4506)
  line L97 (-12.7412, -24.4506) -> (-12.7412, -23.5398)
  line L98 (-12.7412, -23.5398) -> (-11.9075, -23.5398)
  spline S124 degree 2 poles (-6.2419, -20.3133) (-6.2419, -21.4557) (-7.5233, -22.7113) (-8.7068, -22.7113) knots 0 0 0 1 2 2 2
  spline S125 degree 2 poles (-8.7068, -22.7113) (-9.8698, -22.7113) (-11.2489, -21.4917) (-11.2489, -20.5088) knots 0 0 0 1 2 2 2
  spline S126 degree 2 poles (-11.2489, -20.5088) (-11.2489, -20.0663) (-10.9916, -19.3819) (-10.7188, -19.1298) knots 0 0 0 1 2 2 2
  spline S127 degree 2 poles (-10.7188, -19.1298) (-10.4461, -18.8725) (-9.6588, -18.5997) (-9.0876, -18.5997) knots 0 0 0 1 2 2 2
  line L99 (-9.0876, -18.5997) -> (-8.6502, -18.5997)
  line L100 (-8.6502, -18.5997) -> (-8.6502, -21.8982)
  spline S128 degree 2 poles (-8.6502, -21.8982) (-7.8217, -21.8982) (-6.9418, -21.0646) (-6.9418, -20.3236) knots 0 0 0 1 2 2 2
  spline S129 degree 2 poles (-6.9418, -20.3236) (-6.9418, -20.0612) (-7.0601, -19.5517) (-7.1528, -19.3459) knots 0 0 0 1 2 2 2
  spline S130 degree 2 poles (-7.1528, -19.3459) (-7.2557, -19.1298) (-7.4358, -18.8313) (-7.5181, -18.7335) knots 0 0 0 1 2 2 2
  line L101 (-7.5181, -18.7335) -> (-7.5181, -18.6872)
  line L102 (-7.5181, -18.6872) -> (-6.6433, -18.6872)
  spline S131 degree 2 poles (-6.6433, -18.6872) (-6.5867, -18.8262) (-6.422, -19.2481) (-6.3757, -19.4128) knots 0 0 0 1 2 2 2
  spline S132 degree 2 poles (-6.3757, -19.4128) (-6.3088, -19.6443) (-6.2419, -20.0251) (-6.2419, -20.3133) knots 0 0 0 1 2 2 2
  spline S133 degree 2 poles (-9.2626, -19.3819) (-9.5868, -19.3922) (-10.0602, -19.526) (-10.2197, -19.6546) knots 0 0 0 1 2 2 2
  spline S134 degree 2 poles (-10.2197, -19.6546) (-10.3998, -19.7936) (-10.5902, -20.231) (-10.5902, -20.5552) knots 0 0 0 1 2 2 2
  spline S135 degree 2 poles (-10.5902, -20.5552) (-10.5902, -20.8742) (-10.3998, -21.3219) (-10.2145, -21.5071) knots 0 0 0 1 2 2 2
  spline S136 degree 2 poles (-10.2145, -21.5071) (-10.0241, -21.6873) (-9.5662, -21.8725) (-9.2626, -21.8982) knots 0 0 0 1 2 2 2
  line L103 (-9.2626, -21.8982) -> (-9.2626, -19.3819)
  spline S137 degree 2 poles (-6.2419, -15.893) (-6.2419, -16.387) (-6.5455, -17.2052) (-6.8543, -17.4985) knots 0 0 0 1 2 2 2
  spline S138 degree 2 poles (-6.8543, -17.4985) (-7.1579, -17.7918) (-8.0944, -18.116) (-8.7222, -18.116) knots 0 0 0 1 2 2 2
  spline S139 degree 2 poles (-8.7222, -18.116) (-9.35, -18.116) (-10.266, -17.7815) (-10.5748, -17.4985) knots 0 0 0 1 2 2 2
  spline S140 degree 2 poles (-10.5748, -17.4985) (-10.8887, -17.2155) (-11.2231, -16.3767) (-11.2231, -15.893) knots 0 0 0 1 2 2 2
  spline S141 degree 2 poles (-11.2231, -15.893) (-11.2231, -15.5019) (-11.0019, -14.7712) (-10.8578, -14.4882) knots 0 0 0 1 2 2 2
  line L104 (-10.8578, -14.4882) -> (-9.9573, -14.4882)
  line L105 (-9.9573, -14.4882) -> (-9.9573, -14.5345)
  spline S142 degree 2 poles (-9.9573, -14.5345) (-10.0293, -14.622) (-10.2145, -14.8896) (-10.3123, -15.08) knots 0 0 0 1 2 2 2
  spline S143 degree 2 poles (-10.3123, -15.08) (-10.3947, -15.2498) (-10.5233, -15.7026) (-10.5233, -15.9084) knots 0 0 0 1 2 2 2
  spline S144 degree 2 poles (-10.5233, -15.9084) (-10.5233, -16.5311) (-9.5816, -17.2875) (-8.7222, -17.2875) knots 0 0 0 1 2 2 2
  spline S145 degree 2 poles (-8.7222, -17.2875) (-7.8835, -17.2875) (-6.9418, -16.5568) (-6.9418, -15.9084) knots 0 0 0 1 2 2 2
  spline S146 degree 2 poles (-6.9418, -15.9084) (-6.9418, -15.5174) (-7.266, -14.8072) (-7.5181, -14.5345) knots 0 0 0 1 2 2 2
  line L106 (-7.5181, -14.5345) -> (-7.5181, -14.4882)
  line L107 (-7.5181, -14.4882) -> (-6.6176, -14.4882)
  spline S147 degree 2 poles (-6.6176, -14.4882) (-6.561, -14.6065) (-6.4015, -14.9667) (-6.3654, -15.1108) knots 0 0 0 1 2 2 2
  spline S148 degree 2 poles (-6.3654, -15.1108) (-6.3037, -15.3167) (-6.2419, -15.6409) (-6.2419, -15.893) knots 0 0 0 1 2 2 2
  spline S149 degree 2 poles (-6.2574, -12.3166) (-6.2574, -12.9702) (-7.0035, -13.706) (-7.8114, -13.706) knots 0 0 0 1 2 2 2
  line L108 (-7.8114, -13.706) -> (-10.4513, -13.706)
  line L109 (-10.4513, -13.706) -> (-10.4513, -14.2463)
  line L110 (-10.4513, -14.2463) -> (-11.1151, -14.2463)
  line L111 (-11.1151, -14.2463) -> (-11.1151, -13.706)
  line L112 (-11.1151, -13.706) -> (-12.4839, -13.706)
  line L113 (-12.4839, -13.706) -> (-12.4839, -12.9033)
  line L114 (-12.4839, -12.9033) -> (-11.1151, -12.9033)
  line L115 (-11.1151, -12.9033) -> (-11.1151, -11.4264)
  line L116 (-11.1151, -11.4264) -> (-10.4513, -11.4264)
  line L117 (-10.4513, -11.4264) -> (-10.4513, -12.9033)
  line L118 (-10.4513, -12.9033) -> (-8.1819, -12.9033)
  spline S150 degree 2 poles (-8.1819, -12.9033) (-7.8217, -12.9033) (-7.4255, -12.8775) (-7.2557, -12.79) knots 0 0 0 1 2 2 2
  spline S151 degree 2 poles (-7.2557, -12.79) (-7.1064, -12.718) (-6.9572, -12.3938) (-6.9572, -12.1159) knots 0 0 0 1 2 2 2
  spline S152 degree 2 poles (-6.9572, -12.1159) (-6.9572, -11.9204) (-7.0756, -11.555) (-7.1116, -11.4727) knots 0 0 0 1 2 2 2
  line L119 (-7.1116, -11.4727) -> (-7.1116, -11.4264)
  line L120 (-7.1116, -11.4264) -> (-6.3912, -11.4264)
  spline S153 degree 2 poles (-6.3912, -11.4264) (-6.3294, -11.6528) (-6.2574, -12.1159) (-6.2574, -12.3166) knots 0 0 0 1 2 2 2
  spline S154 degree 2 poles (-6.2368, -9.5482) (-6.2368, -10.0267) (-6.4941, -10.8552) (-6.6382, -11.1279) knots 0 0 0 1 2 2 2
  line L121 (-6.6382, -11.1279) -> (-7.5387, -11.1279)
  line L122 (-7.5387, -11.1279) -> (-7.5387, -11.0868)
  spline S155 degree 2 poles (-7.5387, -11.0868) (-7.4564, -10.9838) (-7.2608, -10.706) (-7.1528, -10.4744) knots 0 0 0 1 2 2 2
  spline S156 degree 2 poles (-7.1528, -10.4744) (-7.055, -10.2737) (-6.9109, -9.7797) (-6.9109, -9.5173) knots 0 0 0 1 2 2 2
  spline S157 degree 2 poles (-6.9109, -9.5173) (-6.9109, -9.3269) (-6.9984, -8.8895) (-7.0704, -8.7866) knots 0 0 0 1 2 2 2
  spline S158 degree 2 poles (-7.0704, -8.7866) (-7.1682, -8.6373) (-7.3895, -8.5035) (-7.6159, -8.5035) knots 0 0 0 1 2 2 2
  spline S159 degree 2 poles (-7.6159, -8.5035) (-7.8989, -8.5035) (-8.1922, -8.8123) (-8.29, -9.2085) knots 0 0 0 1 2 2 2
  spline S160 degree 2 poles (-8.29, -9.2085) (-8.326, -9.3629) (-8.4289, -9.8569) (-8.4855, -10.0679) knots 0 0 0 1 2 2 2
  spline S161 degree 2 poles (-8.4855, -10.0679) (-8.6451, -10.6133) (-9.3037, -11.1073) (-9.772, -11.1073) knots 0 0 0 1 2 2 2
  spline S162 degree 2 poles (-9.772, -11.1073) (-10.4204, -11.1073) (-11.2283, -10.1348) (-11.2283, -9.332) knots 0 0 0 1 2 2 2
  spline S163 degree 2 poles (-11.2283, -9.332) (-11.2283, -8.9358) (-11.0327, -8.133) (-10.8835, -7.8603) knots 0 0 0 1 2 2 2
  line L123 (-10.8835, -7.8603) -> (-10.0241, -7.8603)
  line L124 (-10.0241, -7.8603) -> (-10.0241, -7.9015)
  spline S164 degree 2 poles (-10.0241, -7.9015) (-10.2712, -8.2102) (-10.5542, -8.9615) (-10.5542, -9.3475) knots 0 0 0 1 2 2 2
  spline S165 degree 2 poles (-10.5542, -9.3475) (-10.5542, -9.7437) (-10.2197, -10.2892) (-9.8852, -10.2892) knots 0 0 0 1 2 2 2
  spline S166 degree 2 poles (-9.8852, -10.2892) (-9.5816, -10.2892) (-9.2883, -9.965) (-9.1957, -9.6048) knots 0 0 0 1 2 2 2
  spline S167 degree 2 poles (-9.1957, -9.6048) (-9.1494, -9.4298) (-9.0567, -8.9873) (-9.0001, -8.7454) knots 0 0 0 1 2 2 2
  spline S168 degree 2 poles (-9.0001, -8.7454) (-8.8663, -8.2205) (-8.254, -7.6853) (-7.7239, -7.6853) knots 0 0 0 1 2 2 2
  spline S169 degree 2 poles (-7.7239, -7.6853) (-7.4152, -7.6853) (-6.8697, -7.9272) (-6.669, -8.1639) knots 0 0 0 1 2 2 2
  spline S170 degree 2 poles (-6.669, -8.1639) (-6.4581, -8.4161) (-6.2368, -9.0593) (-6.2368, -9.5482) knots 0 0 0 1 2 2 2
  line L125 (-4.9709, -4.0935) -> (-4.9709, -4.814)
  line L126 (-4.9709, -4.814) -> (-12.983, -7.2994)
  line L127 (-12.983, -7.2994) -> (-12.983, -6.5687)
  line L128 (-12.983, -6.5687) -> (-4.9709, -4.0935)
  line L129 (-6.35, -2.0558) -> (-11.9487, -2.0558)
  line L130 (-11.9487, -2.0558) -> (-11.9487, -4.1862)
  line L131 (-11.9487, -4.1862) -> (-12.7, -4.1862)
  line L132 (-12.7, -4.1862) -> (-12.7, 0.9185)
  line L133 (-12.7, 0.9185) -> (-11.9487, 0.9185)
  line L134 (-11.9487, 0.9185) -> (-11.9487, -1.2118)
  line L135 (-11.9487, -1.2118) -> (-6.35, -1.2118)
  line L136 (-6.35, -1.2118) -> (-6.35, -2.0558)
  spline S171 degree 2 poles (-6.2419, 3.5738) (-6.2419, 2.4314) (-7.5233, 1.1758) (-8.7068, 1.1758) knots 0 0 0 1 2 2 2
  spline S172 degree 2 poles (-8.7068, 1.1758) (-9.8698, 1.1758) (-11.2489, 2.3954) (-11.2489, 3.3783) knots 0 0 0 1 2 2 2
  spline S173 degree 2 poles (-11.2489, 3.3783) (-11.2489, 3.8208) (-10.9916, 4.5052) (-10.7188, 4.7574) knots 0 0 0 1 2 2 2
  spline S174 degree 2 poles (-10.7188, 4.7574) (-10.4461, 5.0147) (-9.6588, 5.2874) (-9.0876, 5.2874) knots 0 0 0 1 2 2 2
  line L137 (-9.0876, 5.2874) -> (-8.6502, 5.2874)
  line L138 (-8.6502, 5.2874) -> (-8.6502, 1.9889)
  spline S175 degree 2 poles (-8.6502, 1.9889) (-7.8217, 1.9889) (-6.9418, 2.8225) (-6.9418, 3.5635) knots 0 0 0 1 2 2 2
  spline S176 degree 2 poles (-6.9418, 3.5635) (-6.9418, 3.826) (-7.0601, 4.3354) (-7.1528, 4.5412) knots 0 0 0 1 2 2 2
  spline S177 degree 2 poles (-7.1528, 4.5412) (-7.2557, 4.7574) (-7.4358, 5.0558) (-7.5181, 5.1536) knots 0 0 0 1 2 2 2
  line L139 (-7.5181, 5.1536) -> (-7.5181, 5.1999)
  line L140 (-7.5181, 5.1999) -> (-6.6433, 5.1999)
  spline S178 degree 2 poles (-6.6433, 5.1999) (-6.5867, 5.061) (-6.422, 4.639) (-6.3757, 4.4743) knots 0 0 0 1 2 2 2
  spline S179 degree 2 poles (-6.3757, 4.4743) (-6.3088, 4.2428) (-6.2419, 3.862) (-6.2419, 3.5738) knots 0 0 0 1 2 2 2
  spline S180 degree 2 poles (-9.2626, 4.5052) (-9.5868, 4.4949) (-10.0602, 4.3611) (-10.2197, 4.2325) knots 0 0 0 1 2 2 2
  spline S181 degree 2 poles (-10.2197, 4.2325) (-10.3998, 4.0935) (-10.5902, 3.6561) (-10.5902, 3.332) knots 0 0 0 1 2 2 2
  spline S182 degree 2 poles (-10.5902, 3.332) (-10.5902, 3.0129) (-10.3998, 2.5652) (-10.2145, 2.38) knots 0 0 0 1 2 2 2
  spline S183 degree 2 poles (-10.2145, 2.38) (-10.0241, 2.1999) (-9.5662, 2.0146) (-9.2626, 1.9889) knots 0 0 0 1 2 2 2
  line L141 (-9.2626, 1.9889) -> (-9.2626, 4.5052)
  line L142 (-6.35, 6.9186) -> (-6.35, 6.1159)
  line L143 (-6.35, 6.1159) -> (-12.983, 6.1159)
  line L144 (-12.983, 6.1159) -> (-12.983, 6.9186)
  line L145 (-12.983, 6.9186) -> (-6.35, 6.9186)
  spline S184 degree 2 poles (-6.2419, 10.1657) (-6.2419, 9.0233) (-7.5233, 7.7677) (-8.7068, 7.7677) knots 0 0 0 1 2 2 2
  spline S185 degree 2 poles (-8.7068, 7.7677) (-9.8698, 7.7677) (-11.2489, 8.9873) (-11.2489, 9.9701) knots 0 0 0 1 2 2 2
  spline S186 degree 2 poles (-11.2489, 9.9701) (-11.2489, 10.4127) (-10.9916, 11.0971) (-10.7188, 11.3492) knots 0 0 0 1 2 2 2
  spline S187 degree 2 poles (-10.7188, 11.3492) (-10.4461, 11.6065) (-9.6588, 11.8792) (-9.0876, 11.8792) knots 0 0 0 1 2 2 2
  line L146 (-9.0876, 11.8792) -> (-8.6502, 11.8792)
  line L147 (-8.6502, 11.8792) -> (-8.6502, 8.5807)
  spline S188 degree 2 poles (-8.6502, 8.5807) (-7.8217, 8.5807) (-6.9418, 9.4144) (-6.9418, 10.1554) knots 0 0 0 1 2 2 2
  spline S189 degree 2 poles (-6.9418, 10.1554) (-6.9418, 10.4178) (-7.0601, 10.9273) (-7.1528, 11.1331) knots 0 0 0 1 2 2 2
  spline S190 degree 2 poles (-7.1528, 11.1331) (-7.2557, 11.3492) (-7.4358, 11.6477) (-7.5181, 11.7454) knots 0 0 0 1 2 2 2
  line L148 (-7.5181, 11.7454) -> (-7.5181, 11.7918)
  line L149 (-7.5181, 11.7918) -> (-6.6433, 11.7918)
  spline S191 degree 2 poles (-6.6433, 11.7918) (-6.5867, 11.6528) (-6.422, 11.2309) (-6.3757, 11.0662) knots 0 0 0 1 2 2 2
  spline S192 degree 2 poles (-6.3757, 11.0662) (-6.3088, 10.8346) (-6.2419, 10.4538) (-6.2419, 10.1657) knots 0 0 0 1 2 2 2
  spline S193 degree 2 poles (-9.2626, 11.0971) (-9.5868, 11.0868) (-10.0602, 10.953) (-10.2197, 10.8243) knots 0 0 0 1 2 2 2
  spline S194 degree 2 poles (-10.2197, 10.8243) (-10.3998, 10.6854) (-10.5902, 10.248) (-10.5902, 9.9238) knots 0 0 0 1 2 2 2
  spline S195 degree 2 poles (-10.5902, 9.9238) (-10.5902, 9.6048) (-10.3998, 9.1571) (-10.2145, 8.9718) knots 0 0 0 1 2 2 2
  spline S196 degree 2 poles (-10.2145, 8.9718) (-10.0241, 8.7917) (-9.5662, 8.6065) (-9.2626, 8.5807) knots 0 0 0 1 2 2 2
  line L150 (-9.2626, 8.5807) -> (-9.2626, 11.0971)
  spline S197 degree 2 poles (-6.2368, 13.9788) (-6.2368, 13.5002) (-6.4941, 12.6717) (-6.6382, 12.399) knots 0 0 0 1 2 2 2
  line L151 (-6.6382, 12.399) -> (-7.5387, 12.399)
  line L152 (-7.5387, 12.399) -> (-7.5387, 12.4401)
  spline S198 degree 2 poles (-7.5387, 12.4401) (-7.4564, 12.5431) (-7.2608, 12.8209) (-7.1528, 13.0525) knots 0 0 0 1 2 2 2
  spline S199 degree 2 poles (-7.1528, 13.0525) (-7.055, 13.2532) (-6.9109, 13.7472) (-6.9109, 14.0096) knots 0 0 0 1 2 2 2
  spline S200 degree 2 poles (-6.9109, 14.0096) (-6.9109, 14.2) (-6.9984, 14.6374) (-7.0704, 14.7403) knots 0 0 0 1 2 2 2
  spline S201 degree 2 poles (-7.0704, 14.7403) (-7.1682, 14.8896) (-7.3895, 15.0234) (-7.6159, 15.0234) knots 0 0 0 1 2 2 2
  spline S202 degree 2 poles (-7.6159, 15.0234) (-7.8989, 15.0234) (-8.1922, 14.7146) (-8.29, 14.3184) knots 0 0 0 1 2 2 2
  spline S203 degree 2 poles (-8.29, 14.3184) (-8.326, 14.164) (-8.4289, 13.67) (-8.4855, 13.459) knots 0 0 0 1 2 2 2
  spline S204 degree 2 poles (-8.4855, 13.459) (-8.6451, 12.9136) (-9.3037, 12.4196) (-9.772, 12.4196) knots 0 0 0 1 2 2 2
  spline S205 degree 2 poles (-9.772, 12.4196) (-10.4204, 12.4196) (-11.2283, 13.3921) (-11.2283, 14.1949) knots 0 0 0 1 2 2 2
  spline S206 degree 2 poles (-11.2283, 14.1949) (-11.2283, 14.5911) (-11.0327, 15.3939) (-10.8835, 15.6666) knots 0 0 0 1 2 2 2
  line L153 (-10.8835, 15.6666) -> (-10.0241, 15.6666)
  line L154 (-10.0241, 15.6666) -> (-10.0241, 15.6254)
  spline S207 degree 2 poles (-10.0241, 15.6254) (-10.2712, 15.3167) (-10.5542, 14.5654) (-10.5542, 14.1794) knots 0 0 0 1 2 2 2
  spline S208 degree 2 poles (-10.5542, 14.1794) (-10.5542, 13.7832) (-10.2197, 13.2377) (-9.8852, 13.2377) knots 0 0 0 1 2 2 2
  spline S209 degree 2 poles (-9.8852, 13.2377) (-9.5816, 13.2377) (-9.2883, 13.5619) (-9.1957, 13.9221) knots 0 0 0 1 2 2 2
  spline S210 degree 2 poles (-9.1957, 13.9221) (-9.1494, 14.0971) (-9.0567, 14.5397) (-9.0001, 14.7815) knots 0 0 0 1 2 2 2
  spline S211 degree 2 poles (-9.0001, 14.7815) (-8.8663, 15.3064) (-8.254, 15.8416) (-7.7239, 15.8416) knots 0 0 0 1 2 2 2
  spline S212 degree 2 poles (-7.7239, 15.8416) (-7.4152, 15.8416) (-6.8697, 15.5997) (-6.669, 15.363) knots 0 0 0 1 2 2 2
  spline S213 degree 2 poles (-6.669, 15.363) (-6.4581, 15.1108) (-6.2368, 14.4676) (-6.2368, 13.9788) knots 0 0 0 1 2 2 2
  spline S214 degree 2 poles (-6.2419, 18.4814) (-6.2419, 17.9874) (-6.5455, 17.1692) (-6.8543, 16.8759) knots 0 0 0 1 2 2 2
  spline S215 degree 2 poles (-6.8543, 16.8759) (-7.1579, 16.5826) (-8.0944, 16.2584) (-8.7222, 16.2584) knots 0 0 0 1 2 2 2
  spline S216 degree 2 poles (-8.7222, 16.2584) (-9.35, 16.2584) (-10.266, 16.5929) (-10.5748, 16.8759) knots 0 0 0 1 2 2 2
  spline S217 degree 2 poles (-10.5748, 16.8759) (-10.8887, 17.1589) (-11.2231, 17.9977) (-11.2231, 18.4814) knots 0 0 0 1 2 2 2
  spline S218 degree 2 poles (-11.2231, 18.4814) (-11.2231, 18.8725) (-11.0019, 19.6032) (-10.8578, 19.8862) knots 0 0 0 1 2 2 2
  line L155 (-10.8578, 19.8862) -> (-9.9573, 19.8862)
  line L156 (-9.9573, 19.8862) -> (-9.9573, 19.8399)
  spline S219 degree 2 poles (-9.9573, 19.8399) (-10.0293, 19.7524) (-10.2145, 19.4848) (-10.3123, 19.2944) knots 0 0 0 1 2 2 2
  spline S220 degree 2 poles (-10.3123, 19.2944) (-10.3947, 19.1246) (-10.5233, 18.6718) (-10.5233, 18.4659) knots 0 0 0 1 2 2 2
  spline S221 degree 2 poles (-10.5233, 18.4659) (-10.5233, 17.8433) (-9.5816, 17.0869) (-8.7222, 17.0869) knots 0 0 0 1 2 2 2
  spline S222 degree 2 poles (-8.7222, 17.0869) (-7.8835, 17.0869) (-6.9418, 17.8176) (-6.9418, 18.4659) knots 0 0 0 1 2 2 2
  spline S223 degree 2 poles (-6.9418, 18.4659) (-6.9418, 18.857) (-7.266, 19.5672) (-7.5181, 19.8399) knots 0 0 0 1 2 2 2
  line L157 (-7.5181, 19.8399) -> (-7.5181, 19.8862)
  line L158 (-7.5181, 19.8862) -> (-6.6176, 19.8862)
  spline S224 degree 2 poles (-6.6176, 19.8862) (-6.561, 19.7679) (-6.4015, 19.4076) (-6.3654, 19.2636) knots 0 0 0 1 2 2 2
  spline S225 degree 2 poles (-6.3654, 19.2636) (-6.3037, 19.0577) (-6.2419, 18.7335) (-6.2419, 18.4814) knots 0 0 0 1 2 2 2
  spline S226 degree 2 poles (-8.7325, 24.5329) (-7.5284, 24.5329) (-6.2162, 23.3751) (-6.2162, 22.4077) knots 0 0 0 1 2 2 2
  spline S227 degree 2 poles (-6.2162, 22.4077) (-6.2162, 21.4145) (-7.5696, 20.2773) (-8.7325, 20.2773) knots 0 0 0 1 2 2 2
  spline S228 degree 2 poles (-8.7325, 20.2773) (-9.9264, 20.2773) (-11.2489, 21.4505) (-11.2489, 22.4077) knots 0 0 0 1 2 2 2
  spline S229 degree 2 poles (-11.2489, 22.4077) (-11.2489, 23.3751) (-9.9315, 24.5329) (-8.7325, 24.5329) knots 0 0 0 1 2 2 2
  spline S230 degree 2 poles (-8.7325, 23.7044) (-9.6588, 23.7044) (-10.5593, 23.0303) (-10.5593, 22.4077) knots 0 0 0 1 2 2 2
  spline S231 degree 2 poles (-10.5593, 22.4077) (-10.5593, 21.785) (-9.6588, 21.1058) (-8.7325, 21.1058) knots 0 0 0 1 2 2 2
  spline S232 degree 2 poles (-8.7325, 21.1058) (-7.832, 21.1058) (-6.9058, 21.785) (-6.9058, 22.4077) knots 0 0 0 1 2 2 2
  spline S233 degree 2 poles (-6.9058, 22.4077) (-6.9058, 23.0252) (-7.8166, 23.7044) (-8.7325, 23.7044) knots 0 0 0 1 2 2 2
  spline S234 degree 2 poles (-8.8612, 29.3495) (-7.6673, 29.3495) (-6.2574, 28.2122) (-6.2574, 27.3426) knots 0 0 0 1 2 2 2
  spline S235 degree 2 poles (-6.2574, 27.3426) (-6.2574, 26.9875) (-6.422, 26.442) (-6.5919, 26.159) knots 0 0 0 1 2 2 2
  line L159 (-6.5919, 26.159) -> (-4.5953, 26.159)
  line L160 (-4.5953, 26.159) -> (-4.5953, 25.3563)
  line L161 (-4.5953, 25.3563) -> (-11.1151, 25.3563)
  line L162 (-11.1151, 25.3563) -> (-11.1151, 26.159)
  line L163 (-11.1151, 26.159) -> (-10.6159, 26.159)
  spline S236 degree 2 poles (-10.6159, 26.159) (-10.8887, 26.4575) (-11.2489, 27.1882) (-11.2489, 27.6153) knots 0 0 0 1 2 2 2
  spline S237 degree 2 poles (-11.2489, 27.6153) (-11.2489, 28.4335) (-9.9521, 29.3495) (-8.8612, 29.3495) knots 0 0 0 1 2 2 2
  spline S238 degree 2 poles (-8.7686, 28.521) (-9.5868, 28.521) (-10.4873, 28.0012) (-10.4873, 27.4198) knots 0 0 0 1 2 2 2
  spline S239 degree 2 poles (-10.4873, 27.4198) (-10.4873, 27.0801) (-10.1837, 26.442) (-9.947, 26.159) knots 0 0 0 1 2 2 2
  line L164 (-9.947, 26.159) -> (-7.2402, 26.159)
  spline S240 degree 2 poles (-7.2402, 26.159) (-7.091, 26.4729) (-6.9778, 26.9206) (-6.9778, 27.2088) knots 0 0 0 1 2 2 2
  spline S241 degree 2 poles (-6.9778, 27.2088) (-6.9778, 27.8314) (-7.8938, 28.521) (-8.7686, 28.521) knots 0 0 0 1 2 2 2
  spline S242 degree 2 poles (-6.2419, 32.2517) (-6.2419, 31.1093) (-7.5233, 29.8538) (-8.7068, 29.8538) knots 0 0 0 1 2 2 2
  spline S243 degree 2 poles (-8.7068, 29.8538) (-9.8698, 29.8538) (-11.2489, 31.0733) (-11.2489, 32.0562) knots 0 0 0 1 2 2 2
  spline S244 degree 2 poles (-11.2489, 32.0562) (-11.2489, 32.4987) (-10.9916, 33.1831) (-10.7188, 33.4353) knots 0 0 0 1 2 2 2
  spline S245 degree 2 poles (-10.7188, 33.4353) (-10.4461, 33.6926) (-9.6588, 33.9653) (-9.0876, 33.9653) knots 0 0 0 1 2 2 2
  line L165 (-9.0876, 33.9653) -> (-8.6502, 33.9653)
  line L166 (-8.6502, 33.9653) -> (-8.6502, 30.6668)
  spline S246 degree 2 poles (-8.6502, 30.6668) (-7.8217, 30.6668) (-6.9418, 31.5004) (-6.9418, 32.2414) knots 0 0 0 1 2 2 2
  spline S247 degree 2 poles (-6.9418, 32.2414) (-6.9418, 32.5039) (-7.0601, 33.0133) (-7.1528, 33.2191) knots 0 0 0 1 2 2 2
  spline S248 degree 2 poles (-7.1528, 33.2191) (-7.2557, 33.4353) (-7.4358, 33.7337) (-7.5181, 33.8315) knots 0 0 0 1 2 2 2
  line L167 (-7.5181, 33.8315) -> (-7.5181, 33.8778)
  line L168 (-7.5181, 33.8778) -> (-6.6433, 33.8778)
  spline S249 degree 2 poles (-6.6433, 33.8778) (-6.5867, 33.7389) (-6.422, 33.3169) (-6.3757, 33.1523) knots 0 0 0 1 2 2 2
  spline S250 degree 2 poles (-6.3757, 33.1523) (-6.3088, 32.9207) (-6.2419, 32.5399) (-6.2419, 32.2517) knots 0 0 0 1 2 2 2
  spline S251 degree 2 poles (-9.2626, 33.1831) (-9.5868, 33.1728) (-10.0602, 33.039) (-10.2197, 32.9104) knots 0 0 0 1 2 2 2
  spline S252 degree 2 poles (-10.2197, 32.9104) (-10.3998, 32.7715) (-10.5902, 32.3341) (-10.5902, 32.0099) knots 0 0 0 1 2 2 2
  spline S253 degree 2 poles (-10.5902, 32.0099) (-10.5902, 31.6908) (-10.3998, 31.2431) (-10.2145, 31.0579) knots 0 0 0 1 2 2 2
  spline S254 degree 2 poles (-10.2145, 31.0579) (-10.0241, 30.8778) (-9.5662, 30.6925) (-9.2626, 30.6668) knots 0 0 0 1 2 2 2
  line L169 (-9.2626, 30.6668) -> (-9.2626, 33.1831)
  line L170 (-6.35, 40.2844) -> (-6.35, 39.4405)
  line L171 (-6.35, 39.4405) -> (-11.8201, 39.4405)
  line L172 (-11.8201, 39.4405) -> (-8.0996, 37.7835)
  line L173 (-8.0996, 37.7835) -> (-8.0996, 37.2689)
  line L174 (-8.0996, 37.2689) -> (-11.8201, 35.6274)
  line L175 (-11.8201, 35.6274) -> (-6.35, 35.6274)
  line L176 (-6.35, 35.6274) -> (-6.35, 34.8401)
  line L177 (-6.35, 34.8401) -> (-12.7, 34.8401)
  line L178 (-12.7, 34.8401) -> (-12.7, 35.9928)
  line L179 (-12.7, 35.9928) -> (-9.1648, 37.5777)
  line L180 (-9.1648, 37.5777) -> (-12.7, 39.1112)
  line L181 (-12.7, 39.1112) -> (-12.7, 40.2844)
  line L182 (-12.7, 40.2844) -> (-6.35, 40.2844)
  spline S255 degree 2 poles (-8.7325, 45.4251) (-7.5284, 45.4251) (-6.2162, 44.2673) (-6.2162, 43.2999) knots 0 0 0 1 2 2 2
  spline S256 degree 2 poles (-6.2162, 43.2999) (-6.2162, 42.3067) (-7.5696, 41.1695) (-8.7325, 41.1695) knots 0 0 0 1 2 2 2
  spline S257 degree 2 poles (-8.7325, 41.1695) (-9.9264, 41.1695) (-11.2489, 42.3428) (-11.2489, 43.2999) knots 0 0 0 1 2 2 2
  spline S258 degree 2 poles (-11.2489, 43.2999) (-11.2489, 44.2673) (-9.9315, 45.4251) (-8.7325, 45.4251) knots 0 0 0 1 2 2 2
  spline S259 degree 2 poles (-8.7325, 44.5967) (-9.6588, 44.5967) (-10.5593, 43.9226) (-10.5593, 43.2999) knots 0 0 0 1 2 2 2
  spline S260 degree 2 poles (-10.5593, 43.2999) (-10.5593, 42.6773) (-9.6588, 41.998) (-8.7325, 41.998) knots 0 0 0 1 2 2 2
  spline S261 degree 2 poles (-8.7325, 41.998) (-7.832, 41.998) (-6.9058, 42.6773) (-6.9058, 43.2999) knots 0 0 0 1 2 2 2
  spline S262 degree 2 poles (-6.9058, 43.2999) (-6.9058, 43.9174) (-7.8166, 44.5967) (-8.7325, 44.5967) knots 0 0 0 1 2 2 2
  line L183 (-6.35, 49.9535) -> (-6.35, 49.1508)
  line L184 (-6.35, 49.1508) -> (-6.8749, 49.1508)
  spline S263 degree 2 poles (-6.8749, 49.1508) (-6.5507, 48.7802) (-6.2162, 48.1164) (-6.2162, 47.7048) knots 0 0 0 1 2 2 2
  spline S264 degree 2 poles (-6.2162, 47.7048) (-6.2162, 47.396) (-6.422, 46.8454) (-6.6433, 46.6447) knots 0 0 0 1 2 2 2
  spline S265 degree 2 poles (-6.6433, 46.6447) (-6.8646, 46.4389) (-7.5387, 46.2125) (-8.0224, 46.2125) knots 0 0 0 1 2 2 2
  line L185 (-8.0224, 46.2125) -> (-11.1151, 46.2125)
  line L186 (-11.1151, 46.2125) -> (-11.1151, 47.0152)
  line L187 (-11.1151, 47.0152) -> (-8.3981, 47.0152)
  spline S266 degree 2 poles (-8.3981, 47.0152) (-8.0173, 47.0152) (-7.5181, 47.0718) (-7.3329, 47.1696) knots 0 0 0 1 2 2 2
  spline S267 degree 2 poles (-7.3329, 47.1696) (-7.1476, 47.2674) (-6.9778, 47.6018) (-6.9778, 47.9157) knots 0 0 0 1 2 2 2
  spline S268 degree 2 poles (-6.9778, 47.9157) (-6.9778, 48.2091) (-7.3123, 48.8729) (-7.5541, 49.1508) knots 0 0 0 1 2 2 2
  line L188 (-7.5541, 49.1508) -> (-11.1151, 49.1508)